Autodesk Inventor part; units mm, degrees
(part 8 of 8)
  arc A211 (50.927, 26.2001) -> (50.927, 26.1239) centre (50.927, 26.162) ccw
  arc A212 (51.435, 26.1239) -> (51.435, 26.2001) centre (51.435, 26.162) ccw
  line L104 (53.467, 26.162) -> (53.467, 25.908)
  arc A213 (53.4289, 25.908) -> (53.5051, 25.908) centre (53.467, 25.908) ccw
  arc A214 (53.5051, 26.162) -> (53.4289, 26.162) centre (53.467, 26.162) ccw
  line L105 (53.467, 25.908) -> (53.213, 25.908)
  arc A215 (53.213, 25.9461) -> (53.213, 25.8699) centre (53.213, 25.908) ccw
  arc A216 (53.467, 25.8699) -> (53.467, 25.9461) centre (53.467, 25.908) ccw
  line L106 (53.213, 25.908) -> (53.213, 24.892)
  arc A217 (53.1749, 24.892) -> (53.2511, 24.892) centre (53.213, 24.892) ccw
  arc A218 (53.2511, 25.908) -> (53.1749, 25.908) centre (53.213, 25.908) ccw
  line L107 (53.213, 24.892) -> (53.467, 24.892)
  arc A219 (53.467, 24.8539) -> (53.467, 24.9301) centre (53.467, 24.892) ccw
  arc A220 (53.213, 24.9301) -> (53.213, 24.8539) centre (53.213, 24.892) ccw
  line L108 (53.467, 24.892) -> (53.467, 24.638)
  arc A221 (53.4289, 24.638) -> (53.5051, 24.638) centre (53.467, 24.638) ccw
  arc A222 (53.5051, 24.892) -> (53.4289, 24.892) centre (53.467, 24.892) ccw
  line L109 (53.467, 24.638) -> (53.975, 24.638)
  arc A223 (53.975, 24.5999) -> (53.975, 24.6761) centre (53.975, 24.638) ccw
  arc A224 (53.467, 24.6761) -> (53.467, 24.5999) centre (53.467, 24.638) ccw
  line L110 (53.975, 24.638) -> (53.975, 24.892)
  arc A225 (54.0131, 24.892) -> (53.9369, 24.892) centre (53.975, 24.892) ccw
  arc A226 (53.9369, 24.638) -> (54.0131, 24.638) centre (53.975, 24.638) ccw
  line L111 (53.975, 24.892) -> (54.229, 24.892)
  arc A227 (54.229, 24.8539) -> (54.229, 24.9301) centre (54.229, 24.892) ccw
  arc A228 (53.975, 24.9301) -> (53.975, 24.8539) centre (53.975, 24.892) ccw
  line L112 (54.229, 24.892) -> (54.229, 25.908)
  arc A229 (54.2671, 25.908) -> (54.1909, 25.908) centre (54.229, 25.908) ccw
  arc A230 (54.1909, 24.892) -> (54.2671, 24.892) centre (54.229, 24.892) ccw
  line L113 (54.229, 25.908) -> (53.975, 25.908)
  arc A231 (53.975, 25.9461) -> (53.975, 25.8699) centre (53.975, 25.908) ccw
  arc A232 (54.229, 25.8699) -> (54.229, 25.9461) centre (54.229, 25.908) ccw
  line L114 (53.975, 25.908) -> (53.975, 26.162)
  arc A233 (54.0131, 26.162) -> (53.9369, 26.162) centre (53.975, 26.162) ccw
  arc A234 (53.9369, 25.908) -> (54.0131, 25.908) centre (53.975, 25.908) ccw
  line L115 (53.975, 26.162) -> (53.467, 26.162)
  line L116 (20.574, 24.892) -> (20.828, 24.892)
  arc A235 (53.467, 26.2001) -> (53.467, 26.1239) centre (53.467, 26.162) ccw
  arc A236 (53.975, 26.1239) -> (53.975, 26.2001) centre (53.975, 26.162) ccw
  line L117 (56.007, 26.162) -> (56.007, 25.908)
  arc A237 (55.9689, 25.908) -> (56.0451, 25.908) centre (56.007, 25.908) ccw
  arc A238 (56.0451, 26.162) -> (55.9689, 26.162) centre (56.007, 26.162) ccw
  line L118 (56.007, 25.908) -> (55.753, 25.908)
  arc A239 (55.753, 25.9461) -> (55.753, 25.8699) centre (55.753, 25.908) ccw
  arc A240 (56.007, 25.8699) -> (56.007, 25.9461) centre (56.007, 25.908) ccw
  line L119 (55.753, 25.908) -> (55.753, 24.892)
  arc A241 (55.7149, 24.892) -> (55.7911, 24.892) centre (55.753, 24.892) ccw
  arc A242 (55.7911, 25.908) -> (55.7149, 25.908) centre (55.753, 25.908) ccw
  line L120 (55.753, 24.892) -> (56.007, 24.892)
  arc A243 (56.007, 24.8539) -> (56.007, 24.9301) centre (56.007, 24.892) ccw
  arc A244 (55.753, 24.9301) -> (55.753, 24.8539) centre (55.753, 24.892) ccw
  line L121 (56.007, 24.892) -> (56.007, 24.638)
  arc A245 (55.9689, 24.638) -> (56.0451, 24.638) centre (56.007, 24.638) ccw
  arc A246 (56.0451, 24.892) -> (55.9689, 24.892) centre (56.007, 24.892) ccw
  line L122 (56.007, 24.638) -> (56.515, 24.638)
  arc A247 (56.515, 24.5999) -> (56.515, 24.6761) centre (56.515, 24.638) ccw
  arc A248 (56.007, 24.6761) -> (56.007, 24.5999) centre (56.007, 24.638) ccw
  line L123 (56.515, 24.638) -> (56.515, 24.892)
  arc A249 (56.5531, 24.892) -> (56.4769, 24.892) centre (56.515, 24.892) ccw
  arc A250 (56.4769, 24.638) -> (56.5531, 24.638) centre (56.515, 24.638) ccw
  line L124 (56.515, 24.892) -> (56.769, 24.892)
  arc A251 (56.769, 24.8539) -> (56.769, 24.9301) centre (56.769, 24.892) ccw
  arc A252 (56.515, 24.9301) -> (56.515, 24.8539) centre (56.515, 24.892) ccw
  line L125 (56.769, 24.892) -> (56.769, 25.908)
  arc A253 (56.8071, 25.908) -> (56.7309, 25.908) centre (56.769, 25.908) ccw
  arc A254 (56.7309, 24.892) -> (56.8071, 24.892) centre (56.769, 24.892) ccw
  line L126 (56.769, 25.908) -> (56.515, 25.908)
  arc A255 (56.515, 25.9461) -> (56.515, 25.8699) centre (56.515, 25.908) ccw
  arc A256 (56.769, 25.8699) -> (56.769, 25.9461) centre (56.769, 25.908) ccw
  line L127 (56.515, 25.908) -> (56.515, 26.162)
  arc A257 (56.5531, 26.162) -> (56.4769, 26.162) centre (56.515, 26.162) ccw
  arc A258 (56.4769, 25.908) -> (56.5531, 25.908) centre (56.515, 25.908) ccw
  line L128 (56.515, 26.162) -> (56.007, 26.162)
  arc A259 (56.007, 26.2001) -> (56.007, 26.1239) centre (56.007, 26.162) ccw
  arc A260 (56.515, 26.1239) -> (56.515, 26.2001) centre (56.515, 26.162) ccw
  line L129 (15.748, 25.908) -> (15.494, 25.908)
  arc A261 (15.494, 25.9461) -> (15.494, 25.8699) centre (15.494, 25.908) ccw
  arc A262 (15.748, 25.8699) -> (15.748, 25.9461) centre (15.748, 25.908) ccw
  line L130 (15.494, 25.908) -> (15.494, 26.162)
  arc A263 (15.5321, 26.162) -> (15.4559, 26.162) centre (15.494, 26.162) ccw
  arc A264 (15.4559, 25.908) -> (15.5321, 25.908) centre (15.494, 25.908) ccw
  line L131 (15.494, 26.162) -> (14.986, 26.162)
  arc A265 (14.986, 26.2001) -> (14.986, 26.1239) centre (14.986, 26.162) ccw
  arc A266 (15.494, 26.1239) -> (15.494, 26.2001) centre (15.494, 26.162) ccw
  line L132 (14.986, 26.162) -> (14.986, 25.908)
  arc A267 (14.9479, 25.908) -> (15.0241, 25.908) centre (14.986, 25.908) ccw
  arc A268 (15.0241, 26.162) -> (14.9479, 26.162) centre (14.986, 26.162) ccw
  line L133 (14.986, 25.908) -> (14.732, 25.908)
  arc A269 (14.732, 25.9461) -> (14.732, 25.8699) centre (14.732, 25.908) ccw
  arc A270 (14.986, 25.8699) -> (14.986, 25.9461) centre (14.986, 25.908) ccw
  line L134 (14.732, 25.908) -> (14.732, 24.892)
  arc A271 (14.6939, 24.892) -> (14.7701, 24.892) centre (14.732, 24.892) ccw
  arc A272 (14.7701, 25.908) -> (14.6939, 25.908) centre (14.732, 25.908) ccw
  line L135 (14.732, 24.892) -> (14.986, 24.892)
  arc A273 (20.5359, 24.638) -> (20.6121, 24.638) centre (20.574, 24.638) ccw
  arc A274 (14.986, 24.8539) -> (14.986, 24.9301) centre (14.986, 24.892) ccw
  arc A275 (14.732, 24.9301) -> (14.732, 24.8539) centre (14.732, 24.892) ccw
  line L136 (14.986, 24.892) -> (14.986, 24.638)
  arc A276 (14.9479, 24.638) -> (15.0241, 24.638) centre (14.986, 24.638) ccw
  arc A277 (15.0241, 24.892) -> (14.9479, 24.892) centre (14.986, 24.892) ccw
  line L137 (14.986, 24.638) -> (15.494, 24.638)
  arc A278 (15.494, 24.5999) -> (15.494, 24.6761) centre (15.494, 24.638) ccw
  arc A279 (14.986, 24.6761) -> (14.986, 24.5999) centre (14.986, 24.638) ccw
  line L138 (12.954, 24.638) -> (12.954, 24.892)
  arc A280 (12.9921, 24.892) -> (12.9159, 24.892) centre (12.954, 24.892) ccw
  arc A281 (12.9159, 24.638) -> (12.9921, 24.638) centre (12.954, 24.638) ccw
  line L139 (20.828, 25.908) -> (20.574, 25.908)
  arc A282 (20.574, 25.9461) -> (20.574, 25.8699) centre (20.574, 25.908) ccw
  arc A283 (22.6441, 24.892) -> (22.5679, 24.892) centre (22.606, 24.892) ccw
  arc A284 (20.828, 25.8699) -> (20.828, 25.9461) centre (20.828, 25.908) ccw
  line L140 (20.574, 25.908) -> (20.574, 26.162)
  arc A285 (20.6121, 26.162) -> (20.5359, 26.162) centre (20.574, 26.162) ccw
  arc A286 (20.5359, 25.908) -> (20.6121, 25.908) centre (20.574, 25.908) ccw
  line L141 (20.574, 26.162) -> (20.066, 26.162)
  arc A287 (20.066, 26.2001) -> (20.066, 26.1239) centre (20.066, 26.162) ccw
  arc A288 (20.574, 26.1239) -> (20.574, 26.2001) centre (20.574, 26.162) ccw
  line L142 (20.066, 26.162) -> (20.066, 25.908)
  arc A289 (20.0279, 25.908) -> (20.1041, 25.908) centre (20.066, 25.908) ccw
  arc A290 (20.1041, 26.162) -> (20.0279, 26.162) centre (20.066, 26.162) ccw
  line L143 (20.066, 25.908) -> (19.812, 25.908)
  arc A291 (20.8661, 25.908) -> (20.7899, 25.908) centre (20.828, 25.908) ccw
  arc A292 (19.812, 25.9461) -> (19.812, 25.8699) centre (19.812, 25.908) ccw
  arc A293 (20.066, 25.8699) -> (20.066, 25.9461) centre (20.066, 25.908) ccw
  line L144 (19.812, 25.908) -> (19.812, 24.892)
  arc A294 (19.7739, 24.892) -> (19.8501, 24.892) centre (19.812, 24.892) ccw
  arc A295 (19.8501, 25.908) -> (19.7739, 25.908) centre (19.812, 25.908) ccw
  line L145 (19.812, 24.892) -> (20.066, 24.892)
  arc A296 (20.066, 24.8539) -> (20.066, 24.9301) centre (20.066, 24.892) ccw
  arc A297 (19.812, 24.9301) -> (19.812, 24.8539) centre (19.812, 24.892) ccw
  line L146 (20.066, 24.892) -> (20.066, 24.638)
  arc A298 (20.0279, 24.638) -> (20.1041, 24.638) centre (20.066, 24.638) ccw
  arc A299 (20.1041, 24.892) -> (20.0279, 24.892) centre (20.066, 24.892) ccw
  line L147 (20.066, 24.638) -> (20.574, 24.638)
  arc A300 (20.574, 24.5999) -> (20.574, 24.6761) centre (20.574, 24.638) ccw
  arc A301 (20.066, 24.6761) -> (20.066, 24.5999) centre (20.066, 24.638) ccw
  line L148 (18.034, 24.638) -> (18.034, 24.892)
  arc A302 (18.0721, 24.892) -> (17.9959, 24.892) centre (18.034, 24.892) ccw
  arc A303 (17.9959, 24.638) -> (18.0721, 24.638) centre (18.034, 24.638) ccw
  line L149 (18.034, 24.892) -> (18.288, 24.892)
  arc A304 (18.288, 24.8539) -> (18.288, 24.9301) centre (18.288, 24.892) ccw
  arc A305 (18.034, 24.9301) -> (18.034, 24.8539) centre (18.034, 24.892) ccw
  line L150 (18.288, 24.892) -> (18.288, 25.908)
  arc A306 (18.3261, 25.908) -> (18.2499, 25.908) centre (18.288, 25.908) ccw
  arc A307 (18.2499, 24.892) -> (18.3261, 24.892) centre (18.288, 24.892) ccw
  line L151 (18.288, 25.908) -> (18.034, 25.908)
  arc A308 (18.034, 25.9461) -> (18.034, 25.8699) centre (18.034, 25.908) ccw
  arc A309 (18.288, 25.8699) -> (18.288, 25.9461) centre (18.288, 25.908) ccw
  line L152 (18.034, 25.908) -> (18.034, 26.162)
  arc A310 (18.0721, 26.162) -> (17.9959, 26.162) centre (18.034, 26.162) ccw
  arc A311 (20.6121, 24.892) -> (20.5359, 24.892) centre (20.574, 24.892) ccw
  line L153 (23.114, 24.638) -> (23.114, 24.892)
  constraints: 928 point on circle, 312 centre point, 308 end point, 304 point on line
sketch "Sketch10" plane through (0, 0, 0) normal (0, 0, 1) x (1, 0, 0)
  line L0 (0, 0) -> (110.49, 0)
  line L1 (110.49, 0) -> (110.49, 85.09)
  line L2 (110.49, 85.09) -> (0, 85.09)
  line L3 (0, 85.09) -> (0, 0)
  arc A0 (12.0927, 65.3321) -> (12.0927, 84.3321) centre (12.0927, 74.8321) ccw projected
  arc A1 (12.0927, 84.3321) -> (12.0927, 65.3321) centre (12.0927, 74.8321) ccw projected
  arc A2 (33.5609, 84.4119) -> (33.5609, 65.4119) centre (33.5609, 74.9119) ccw projected
  arc A3 (55.2196, 84.5062) -> (55.2196, 65.5062) centre (55.2196, 75.0062) ccw projected
  arc A4 (76.8576, 84.3321) -> (76.8576, 65.3321) centre (76.8576, 74.8321) ccw projected
  arc A5 (98.4424, 84.3321) -> (98.4424, 65.3321) centre (98.4424, 74.8321) ccw projected
  arc A6 (12.0477, 63.2972) -> (12.0477, 44.2972) centre (12.0477, 53.7972) ccw projected
  arc A7 (33.6842, 63.4569) -> (33.6842, 44.4569) centre (33.6842, 53.9569) ccw projected
  arc A8 (55.2831, 63.3771) -> (55.2831, 44.3771) centre (55.2831, 53.8771) ccw projected
  arc A9 (76.8504, 63.4569) -> (76.8504, 44.4569) centre (76.8504, 53.9569) ccw projected
  arc A10 (98.4424, 63.4569) -> (98.4424, 44.4569) centre (98.4424, 53.9569) ccw projected
  arc A11 (12.085, 21.5469) -> (12.085, 2.5469) centre (12.085, 12.0469) ccw projected
  arc A12 (12.085, 2.5469) -> (12.085, 21.5469) centre (12.085, 12.0469) ccw projected
  arc A13 (33.6796, 21.5886) -> (33.6796, 2.5886) centre (33.6796, 12.0886) ccw projected
  arc A14 (33.6796, 2.5886) -> (33.6796, 21.5886) centre (33.6796, 12.0886) ccw projected
  arc A15 (55.3493, 21.6412) -> (55.3493, 2.6412) centre (55.3493, 12.1412) ccw projected
  arc A16 (55.3493, 2.6412) -> (55.3493, 21.6412) centre (55.3493, 12.1412) ccw projected
  arc A17 (76.942, 21.6412) -> (76.942, 2.6412) centre (76.942, 12.1412) ccw projected
  arc A18 (76.942, 2.6412) -> (76.942, 21.6412) centre (76.942, 12.1412) ccw projected
  arc A19 (98.4424, 21.6412) -> (98.4424, 2.6412) centre (98.4424, 12.1412) ccw projected
  arc A20 (98.4424, 2.6412) -> (98.4424, 21.6412) centre (98.4424, 12.1412) ccw projected
  arc A21 (98.4358, 23.2896) -> (98.4358, 42.2896) centre (98.4358, 32.7896) ccw projected
  arc A22 (98.4358, 42.2896) -> (98.4358, 23.2896) centre (98.4358, 32.7896) ccw projected
  arc A23 (98.4424, 44.4569) -> (98.4424, 63.4569) centre (98.4424, 53.9569) ccw projected
  arc A24 (76.8504, 44.4569) -> (76.8504, 63.4569) centre (76.8504, 53.9569) ccw projected
  arc A25 (55.2831, 44.3771) -> (55.2831, 63.3771) centre (55.2831, 53.8771) ccw projected
  arc A26 (33.6842, 44.4569) -> (33.6842, 63.4569) centre (33.6842, 53.9569) ccw projected
  arc A27 (12.0477, 44.2972) -> (12.0477, 63.2972) centre (12.0477, 53.7972) ccw projected
  arc A28 (33.5609, 65.4119) -> (33.5609, 84.4119) centre (33.5609, 74.9119) ccw projected
  arc A29 (55.2196, 65.5062) -> (55.2196, 84.5062) centre (55.2196, 75.0062) ccw projected
  arc A30 (76.8576, 65.3321) -> (76.8576, 84.3321) centre (76.8576, 74.8321) ccw projected
  arc A31 (98.4424, 65.3321) -> (98.4424, 84.3321) centre (98.4424, 74.8321) ccw projected
  circle A32 centre (22.225, 65.7225) radius 1.524 projected
  circle A33 centre (87.376, 65.7225) radius 1.524 projected
  circle A34 centre (87.376, 19.431) radius 1.524 projected
  circle A35 centre (22.225, 19.431) radius 1.524 projected
  line L4 (0, 85.09) -> (110.49, 0) construction
  line L5 (112.99, -2.5) -> (-2.5, -2.5)
  line L6 (-2.5, -2.5) -> (-2.5, 87.59)
  line L7 (-2.5, 87.59) -> (112.99, 87.59)
  line L8 (112.99, 87.59) -> (112.99, -2.5)
  line L9 (112.99, -2.5) -> (-2.5, 87.59) construction
  line L10 (-2.5, -2.5) -> (112.99, 87.59) construction
  line L11 (-5.5, -2.5) -> (115.99, -2.5)
  line L12 (115.99, -2.5) -> (115.99, 90.59)
  line L13 (115.99, 90.59) -> (-5.5, 90.59)
  line L14 (-5.5, 90.59) -> (-5.5, -2.5)
  point P0 (55.245, 42.545)
  point P1 (-2.5, -2.5)
  dimension "d0" = 110.49
  dimension "d1" = 85.09
  dimension "d5" = 2.5
  dimension "d6" = 2.5
  dimension "d7" = 3
  dimension "d8" = 3
  dimension "d9" = 3
  constraints: 30 end point, 6 parallel, 3 horizontal, 3 midpoint, 3 perpendicular, 1 collinear
  measures "d0" distance of L2.end L1.end
  measures "d1" distance of L1.end L0.end
  measures "d5" distance between parallel lines of L7 L2
  measures "d6" distance between parallel lines of L8 L1
  measures "d7" distance between parallel lines of L12 L8
  measures "d8" distance between parallel lines of L13 L7
  measures "d9" distance between parallel lines of L14 L6
extrude "Extrusion1" add sketch "Sketch10" along normal blind 5 contours L3 L2 L1 L0 | L5 L6 L7 L8 | L8 L7 L6 L11 L14 L13 L12
body "Solid1"
